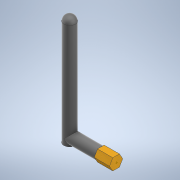
# Autodesk Inventor part: antena
Saved by Autodesk Inventor 2020 (Build 240168000, 168)
## iProperties
Created: 2021-10-19
Part Number: antena
Material: Genérico
Document SubType Name: Modeling
Designer: DANIEL
Density: 1 g/cm^3
Appearance: Valor por defecto
Author: DANIEL
Autodesk Inventor part; units mm, degrees
ref_plane "YZ Plane" through (0, 0, 0) normal (1, 0, 0) x (0, 1, 0)
ref_plane "XZ Plane" through (0, 0, 0) normal (0, 1, 0) x (-1, 0, 0)
ref_plane "XY Plane" through (0, 0, 0) normal (0, 0, 1) x (1, 0, 0)
sketch "Boceto1" plane through (0, 0, 0) normal (0, 1, 0) x (-1, 0, 0)
  circle A0 centre (0, 0) radius 4.5
  dimension "d0" = 9
  constraints: 1 centre point, 1 coincident
  measures "d0" diameter of A0
extrude "Extrusión1" add sketch "Boceto1" along normal blind 87
fillet "Empalme1" radius 4.5 1 edges at (4.5, 87, 0)
sketch "Boceto2" plane through (0, 0, 0) normal (0, -1, 0) x (1, 0, 0)
  circle A0 centre (0, 0) radius 4.5 projected
  circle A1 centre (0, 0) radius 4.5 projected
  line L0 (3.8723, -2.2357) -> (3.8971, -2.25)
  line L1 (0, 0) -> (5.1962, 0) construction
  line L2 (4.5, -2.5981) -> (4.5, 2.5981)
  line L3 (0, 0) -> (5.1962, 0) construction
  line L4 (4.5, 2.5981) -> (0, 5.1958)
  line L5 (0, 5.1958) -> (-4.5, 2.5981)
  line L6 (-4.5, 2.5981) -> (-4.5409, -2.5978)
  line L7 (-4.5409, -2.5978) -> (-0.0409, -5.1955)
  line L8 (-0.0409, -5.1955) -> (4.5, -2.5981)
  dimension "d9" = 30
  dimension "d11" = 5.196
  dimension "d12" = 5.196
  dimension "d13" = 5.196
  dimension "d14" = 5.196
  constraints: 18 end point, 2 horizontal, 1 parallel, 2 other
  measures "d9" angle of L0 L1
  measures "d11" distance of L2.end L4.end
  measures "d12" distance of L4.end L5.end
  measures "d13" distance of L5.end L6.end
  measures "d14" distance of L6.end L7.end
extrude "Extrusión2" [suppressed]
ref_plane "Plano de trabajo1" through (-2.2861, 0, 1.3081) normal (-0.5, 0, -0.8661) x (-0.8661, 0, 0.5)
ref_plane "Plano de trabajo2" through (4.5, 0, -2.5981) normal (0.5, 0, 0.866) x (0, 1, 0)
sketch "Boceto4" plane through (0, 0, 0) normal (1, 0, 0) x (0, 1, 0)
  circle A0 centre (4.5, 0) radius 4.5
  line L0 (0, -4.5) -> (0, 4.5) projected
  line L1 (0, 4.5) -> (82.5, 4.5) projected
  point P0 (0, 0)
  dimension "d18" = 9
  dimension "d19" = 4.5
  dimension "d20" = 4.5
  constraints: 1 centre point
  measures "d18" diameter of A0
  measures "d19" distance from line of A0.centre L0
  measures "d20" distance from line of L1 A0.centre
extrude "Extrusión3" add sketch "Boceto4" along normal blind 24.5 contours A0
sketch "Boceto5" plane through (24.5, 4.5, 0) normal (1, 0, 0) x (0, 0, -1)
  circle A0 centre (0, 0) radius 4.5 projected
  circle A1 centre (0, 0) radius 4.5
  line L0 (0, 4.5) -> (-2.5981, 4.5)
  line L1 (-2.5981, 4.5) -> (2.5981, 4.5)
  line L2 (0, 4.5) -> (2.5981, 4.5) construction
  line L3 (0, 0) -> (5.9241, 0) construction
  line L4 (0, 0) -> (-9, 0)
  line L5 (0, 0) -> (6.2143, 0) construction
  line L6 (-3.8971, 2.25) -> (-5.1962, 0)
  line L7 (-5.1962, 0) -> (-2.5981, 4.5)
  line L8 (-5.1962, 0) -> (-2.5981, -4.5)
  line L9 (-5.1962, 0) -> (2.2031, 0) construction
  line L10 (4.5, -4.5) -> (-4.5, -4.5) projected
  line L11 (0, -4.5) -> (-2.5981, -4.5)
  line L12 (-4.5, -4.5) -> (2.5981, -4.5)
  line L13 (0, -4.5) -> (2.5981, -4.5)
  line L14 (2.5981, -4.5) -> (5.1096, -0.1499)
  line L15 (5.1096, -0.1499) -> (5.1962, 0)
  line L16 (5.1962, 0) -> (2.5981, 4.5)
  line L17 (5.1962, 0) -> (10.3923, 0) construction
  line L18 (-2.5981, -4.5) -> (-5.1962, 0)
  line L19 (-2.5981, 4.5) -> (2.5981, 4.5)
  dimension "d26" = 60
  dimension "Q" = 2.5981
  dimension "d28" = 2.5981
  dimension "d29" = 120
  constraints: 38 end point, 8 horizontal, 3 point on line, 2 collinear, 2 point on circle, 2 tangent, 1 centre point, 1 coincident, 1 equal length, 1 vertical alignment, 1 other
  measures "d26" angle of L8 L9
  measures "Q" distance of L8.end L11.start
  measures "d28" distance of L12.end L11.start
  measures "d29" angle of L17 L16
extrude "Extrusión4" add sketch "Boceto5" along normal blind 12
equation "\"d28\" = Q"
